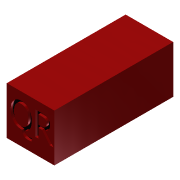
# Autodesk Inventor part: Container 2 2 5 QR color 4
Saved by Autodesk Inventor 2015 (Build 190159000, 159)
## iProperties
Created: 2015-03-07
Part Number: Container 2 2 5 QR color 4
Material: Generic
Document SubType Name: Modeling
Designer: Vukica
Density: 1 g/cm^3
Appearance: Red
Author: Vukica
Autodesk Inventor part; units mm, degrees
ref_plane "YZ Plane" through (0, 0, 0) normal (1, 0, 0) x (0, 1, 0)
ref_plane "XZ Plane" through (0, 0, 0) normal (0, 1, 0) x (-1, 0, 0)
ref_plane "XY Plane" through (0, 0, 0) normal (0, 0, 1) x (1, 0, 0)
sketch "Sketch1" plane through (0, 0, 0) normal (0, 0, 1) x (1, 0, 0)
  line L0 (0, 0) -> (50.8, 0)
  line L1 (50.8, 0) -> (50.8, 50.8)
  line L2 (50.8, 50.8) -> (0, 50.8)
  line L3 (0, 50.8) -> (0, 0)
  dimension "d0" = 50.8
  dimension "d1" = 50.8
  constraints: 8 end point, 2 parallel, 1 horizontal, 1 perpendicular
  measures "d0" distance of L1.end L2.end
  measures "d1" distance of L2.end L0.start
extrude "Extrusion1" add sketch "Sketch1" along normal blind 127
sketch "Sketch2" plane through (0, 0, 127) normal (0, 0, 1) x (1, 0, 0)
  line L0 (3.0193, 42.2087) -> (49.4145, 42.2087) construction
  line L1 (49.4145, 42.2087) -> (49.4145, 9.5839) construction
  line L2 (49.4145, 9.5839) -> (3.0193, 9.5839) construction
  line L3 (3.0193, 9.5839) -> (3.0193, 42.2087) construction
  spline S0 degree 2 poles (26.6903, 10.0573) (25.7641, 9.8309) (23.7469, 9.5839) (22.7383, 9.5839) knots 0 0 0 1 2 2 2
  spline S1 degree 2 poles (22.7383, 9.5839) (19.8772, 9.5839) (16.3162, 12.7743) (16.1516, 15.7383) knots 0 0 0 1 2 2 2
  spline S2 degree 2 poles (16.1516, 15.7383) (15.9252, 15.7383) (15.5341, 15.7383) (15.3694, 15.7383) knots 0 0 0 1 2 2 2
  spline S3 degree 2 poles (15.3694, 15.7383) (12.7965, 15.7383) (8.6592, 17.4879) (7.1772, 19.1964) knots 0 0 0 1 2 2 2
  spline S4 degree 2 poles (7.1772, 19.1964) (5.7158, 20.8842) (4.1514, 25.8242) (4.1514, 28.9529) knots 0 0 0 1 2 2 2
  spline S5 degree 2 poles (4.1514, 28.9529) (4.1514, 32.164) (5.7363, 37.0217) (7.1978, 38.7507) knots 0 0 0 1 2 2 2
  spline S6 degree 2 poles (7.1978, 38.7507) (8.6798, 40.4591) (12.8171, 42.2087) (15.3694, 42.2087) knots 0 0 0 1 2 2 2
  spline S7 degree 2 poles (15.3694, 42.2087) (17.9629, 42.2087) (22.1208, 40.3973) (23.5616, 38.7507) knots 0 0 0 1 2 2 2
  spline S8 degree 2 poles (23.5616, 38.7507) (25.0025, 37.0834) (26.608, 32.1228) (26.608, 28.9529) knots 0 0 0 1 2 2 2
  spline S9 degree 2 poles (26.608, 28.9529) (26.608, 24.0129) (22.7589, 17.5909) (19.4038, 16.4588) knots 0 0 0 1 2 2 2
  spline S10 degree 2 poles (19.4038, 16.4588) (19.4861, 15.5119) (19.9801, 13.9888) (20.3712, 13.5565) knots 0 0 0 1 2 2 2
  spline S11 degree 2 poles (20.3712, 13.5565) (20.8446, 13.0213) (22.1414, 12.5273) (23.294, 12.5273) knots 0 0 0 1 2 2 2
  spline S12 degree 2 poles (23.294, 12.5273) (23.9733, 12.5273) (25.8258, 12.9596) (26.2375, 13.1242) knots 0 0 0 1 2 2 2
  line L4 (26.2375, 13.1242) -> (26.6903, 13.1242)
  line L5 (26.6903, 13.1242) -> (26.6903, 10.0573)
  spline S13 degree 2 poles (23.0882, 28.9529) (23.0882, 31.4847) (21.9973, 35.375) (21.0093, 36.6512) knots 0 0 0 1 2 2 2
  spline S14 degree 2 poles (21.0093, 36.6512) (20.0007, 37.9685) (17.1602, 39.2858) (15.39, 39.2858) knots 0 0 0 1 2 2 2
  spline S15 degree 2 poles (15.39, 39.2858) (13.5581, 39.2858) (10.7999, 38.0097) (9.7501, 36.6512) knots 0 0 0 1 2 2 2
  spline S16 degree 2 poles (9.7501, 36.6512) (8.7415, 35.3544) (7.6712, 31.423) (7.6712, 28.9529) knots 0 0 0 1 2 2 2
  spline S17 degree 2 poles (7.6712, 28.9529) (7.6712, 23.9512) (11.8702, 18.62) (15.39, 18.62) knots 0 0 0 1 2 2 2
  spline S18 degree 2 poles (15.39, 18.62) (18.9098, 18.62) (23.0882, 23.9512) (23.0882, 28.9529) knots 0 0 0 1 2 2 2
  line L6 (49.9702, 16.2735) -> (45.5859, 16.2735)
  line L7 (45.5859, 16.2735) -> (37.5584, 26.38)
  line L8 (37.5584, 26.38) -> (33.6887, 26.38)
  line L9 (33.6887, 26.38) -> (33.6887, 16.2735)
  line L10 (33.6887, 16.2735) -> (30.313, 16.2735)
  line L11 (30.313, 16.2735) -> (30.313, 41.6735)
  line L12 (30.313, 41.6735) -> (36.8586, 41.6735)
  spline S19 degree 2 poles (36.8586, 41.6735) (39.0404, 41.6735) (41.9838, 41.2001) (43.3218, 40.3356) knots 0 0 0 1 2 2 2
  spline S20 degree 2 poles (43.3218, 40.3356) (44.6597, 39.4711) (46.2034, 36.7747) (46.2034, 34.7781) knots 0 0 0 1 2 2 2
  spline S21 degree 2 poles (46.2034, 34.7781) (46.2034, 31.9993) (43.3629, 28.2325) (40.9341, 27.3268) knots 0 0 0 1 2 2 2
  line L13 (40.9341, 27.3268) -> (49.9702, 16.2735)
  spline S22 degree 2 poles (42.6837, 34.5105) (42.6837, 35.622) (41.9015, 37.3304) (41.0782, 37.8862) knots 0 0 0 1 2 2 2
  spline S23 degree 2 poles (41.0782, 37.8862) (40.3577, 38.3596) (38.4435, 38.7507) (37.0438, 38.7507) knots 0 0 0 1 2 2 2
  line L14 (37.0438, 38.7507) -> (33.6887, 38.7507)
  line L15 (33.6887, 38.7507) -> (33.6887, 29.1999)
  line L16 (33.6887, 29.1999) -> (36.6527, 29.1999)
  spline S24 degree 2 poles (36.6527, 29.1999) (38.1141, 29.1999) (40.4401, 29.7145) (41.2428, 30.5173) knots 0 0 0 1 2 2 2
  spline S25 degree 2 poles (41.2428, 30.5173) (41.9838, 31.2171) (42.6837, 33.1931) (42.6837, 34.5105) knots 0 0 0 1 2 2 2
  point P0 (0, 0)
  constraints: 2 other
extrude "Extrusion2" cut sketch "Sketch2" against normal blind 2.54
body "Solid1"
